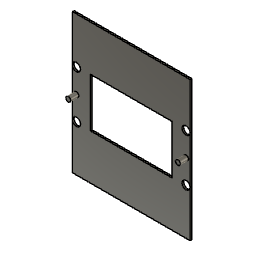
Cube_Plate_Viewing_window (Autodesk Fusion 360 design; units mm, degrees)
Autodesk Fusion 360 part; units mm, degrees
sketch "Esquisse1" plane through (0, 0, 0) normal (0, 1, 0) x (1, 0, 0)
  line L0 (36.115, 26.289) -> (-36.115, 26.289)
  line L1 (-36.115, 26.289) -> (-36.115, -26.289)
  line L2 (-36.115, -26.289) -> (36.115, -26.289)
  line L3 (36.115, -26.289) -> (36.115, 26.289)
  line L4 (36.115, 26.289) -> (-36.115, -26.289) construction
  line L5 (-36.115, 26.289) -> (36.115, -26.289) construction
  line L6 (36.115, 0) -> (31.115, 0) construction
  circle A0 centre (33.615, 0) radius 1.5
  line L7 (33.615, 0) -> (33.615, -14.516) construction
  circle A1 centre (33.615, -14.516) radius 1.5
  circle A2 centre (33.615, 14.516) radius 1.5
  line L8 (0, 0) -> (0, -26.289) construction
  circle A3 centre (-33.615, -14.516) radius 1.5
  circle A4 centre (-33.615, 0) radius 1.5
  circle A5 centre (-33.615, 14.516) radius 1.5
  line L9 (25, 15) -> (-25, 15)
  line L10 (-25, 15) -> (-25, -15)
  line L11 (-25, -15) -> (25, -15)
  line L12 (25, -15) -> (25, 15)
  line L13 (25, 15) -> (-25, -15) construction
  line L14 (-25, 15) -> (25, -15) construction
  dimension "d1" = 72.23
  dimension "d2" = 52.578
  dimension "d5" = 5
  dimension "d6" = 3
  dimension "d7" = 14.516
  dimension "d8" = 3
  dimension "d9" = 50
  dimension "d10" = 30
  constraint horizontal L0
  constraint perpendicular L0 L1
  constraint parallel L0 L2
  constraint parallel L1 L3
  constraint coincident L4 L8.start
  constraint coincident L5 L8.start
  constraint coincident L8.start origin
  constraint midpoint L3 L6.start
  constraint perpendicular L3 L6
  constraint midpoint L6 A0.centre
  constraint coincident A0.centre L7.start
  constraint perpendicular L6 L7
  constraint coincident L7.end A1.centre
  constraint symmetric L6 A1 A2
  constraint midpoint L2 L8.end
  constraint symmetric A0 L8 A4
  constraint symmetric A1 L8 A3
  constraint symmetric A2 L8 A5
  constraint horizontal L9
  constraint perpendicular L9 L10
  constraint parallel L9 L11
  constraint parallel L10 L12
  constraint coincident L13 L8.start
  constraint coincident L14 L8.start
  measures "d1" distance of L1.end L2.end
  measures "d2" distance of L0.end L1.end
  measures "d5" distance of L6.start L6.end
  measures "d6" diameter of A0
  measures "d7" distance of A0.centre L7.end
  measures "d8" diameter of A1
  measures "d9" distance of L10.end L11.end
  measures "d10" distance of L9.end L10.end
extrude "Extrusion1" add sketch "Esquisse1" along normal blind 1 contours L0 L1 L2 L3 | A0 | A4
sketch "Sketch2" plane through (0, 1, 0) normal (0, 1, 0) x (-1, 0, 0)
  line L0 (-25, -15) -> (-25, 15)
  line L1 (-25, 15) -> (25, 15)
  line L2 (25, 15) -> (25, -15)
  line L3 (25, -15) -> (-25, -15)
  circle A0 centre (33.615, 14.516) radius 1.5
  circle A1 centre (33.615, -14.516) radius 1.5
  circle A2 centre (-33.615, -14.516) radius 1.5
  circle A3 centre (-33.615, 14.516) radius 1.5
  line L4 (-36.115, 26.289) -> (-36.115, -26.289)
  line L5 (-36.115, -26.289) -> (36.115, -26.289)
  line L6 (36.115, -26.289) -> (36.115, 26.289)
  line L7 (36.115, 26.289) -> (-36.115, 26.289)
  circle A4 centre (-33.615, 14.516) radius 2.5
  circle A5 centre (33.615, 14.516) radius 2.5
  circle A6 centre (33.615, -14.516) radius 2.5
  circle A7 centre (-33.615, -14.516) radius 2.5
  dimension "d13" = 5
  dimension "d14" = 5
  dimension "d15" = 5
  dimension "d16" = 5
  constraint concentric A3 A4
  constraint concentric A0 A5
  constraint concentric A1 A6
  constraint concentric A2 A7
  measures "d13" diameter of A4
  measures "d14" diameter of A5
  measures "d15" diameter of A6
  measures "d16" diameter of A7
extrude "Extrude3" cut sketch "Sketch2" against normal blind 1 contours A4 | A7 | A6 | A5
extrude "Extrude2" add sketch "Esquisse1" against normal blind 5 contours A0 | A4
extrude "Extrude4" add 1 faces at (-12.0383, 0.6667, 26.289) along direction (0, 0, 1) blind 16.5
extrude "Extrude5" add 1 faces at (12.0383, 0.6667, -26.289) along direction (0, 0, -1) blind 16.5
equation "d2 = 39.032 mm + ( 6.773 * 2 ) * 1 mm"
